Autodesk Fusion 360 part; units mm, degrees
(part 15 of 15)
  spline S61 degree 5 poles (-15.8444, 6.1608) (-15.8425, 6.1587) (-15.8389, 6.1545) (-15.8334, 6.1482) (-15.8261, 6.1398) (-15.8169, 6.1293) (-15.8078, 6.1189) (-15.7986, 6.1086) (-15.7895, 6.0982) (-15.7804, 6.0879) (-15.7712, 6.0777) (-15.7621, 6.0675) (-15.753, 6.0573) (-15.7439, 6.0472) (-15.7347, 6.0371) (-15.7256, 6.027) (-15.7165, 6.017) (-15.7074, 6.007) (-15.6983, 5.9971) (-15.6892, 5.9872) (-15.6801, 5.9774) (-15.671, 5.9676) (-15.6619, 5.9578) (-15.6529, 5.9481) (-15.6438, 5.9384) (-15.6347, 5.9287) (-15.6256, 5.9191) (-15.6166, 5.9096) (-15.6075, 5.9) (-15.5985, 5.8905) (-15.5895, 5.8811) (-15.5804, 5.8717) (-15.5714, 5.8623) (-15.5624, 5.853) (-15.5534, 5.8437) (-15.5444, 5.8345) (-15.5354, 5.8253) (-15.5264, 5.8162) (-15.5174, 5.8071) (-15.5084, 5.798) (-15.4995, 5.789) (-15.4905, 5.78) (-15.4816, 5.771) (-15.4726, 5.7621) (-15.4637, 5.7532) (-15.4548, 5.7444) (-15.4458, 5.7356) (-15.4369, 5.7269) (-15.428, 5.7182) (-15.4192, 5.7096) (-15.4103, 5.7009) (-15.4014, 5.6924) (-15.3926, 5.6838) (-15.3837, 5.6753) (-15.3749, 5.6669) (-15.3661, 5.6585) (-15.3572, 5.6501) (-15.3484, 5.6418) (-15.3397, 5.6335) (-15.3309, 5.6253) (-15.3221, 5.6171) (-15.3134, 5.609) (-15.3046, 5.6008) (-15.2959, 5.5928) (-15.2872, 5.5848) (-15.2785, 5.5768) (-15.2698, 5.5688) (-15.2611, 5.5609) (-15.2524, 5.5531) (-15.2438, 5.5453) (-15.2352, 5.5375) (-15.2265, 5.5298) (-15.2179, 5.5221) (-15.2093, 5.5144) (-15.2008, 5.5068) (-15.1922, 5.4993) (-15.1836, 5.4918) (-15.1751, 5.4843) (-15.1666, 5.4769) (-15.1581, 5.4695) (-15.1496, 5.4621) (-15.1411, 5.4548) (-15.1327, 5.4476) (-15.1242, 5.4403) (-15.1158, 5.4332) (-15.1074, 5.426) (-15.099, 5.419) (-15.0907, 5.4119) (-15.0823, 5.4049) (-15.074, 5.398) (-15.0657, 5.391) (-15.0574, 5.3842) (-15.0491, 5.3773) (-15.0409, 5.3706) (-15.0326, 5.3638) (-15.0244, 5.3571) (-15.0162, 5.3505) (-15.008, 5.3439) (-14.9999, 5.3373) (-14.9918, 5.3308) (-14.9836, 5.3243) (-14.9755, 5.3178) (-14.9675, 5.3114) (-14.9594, 5.3051) (-14.9514, 5.2988) (-14.9434, 5.2925) (-14.9354, 5.2863) (-14.9275, 5.2801) (-14.9195, 5.274) (-14.9116, 5.2679) (-14.9037, 5.2619) (-14.8959, 5.2559) (-14.888, 5.2499) (-14.8802, 5.244) (-14.8724, 5.2381) (-14.8646, 5.2323) (-14.8569, 5.2265) (-14.8492, 5.2208) (-14.8415, 5.2151) (-14.8338, 5.2094) (-14.8262, 5.2038) (-14.8186, 5.1982) (-14.811, 5.1927) (-14.8035, 5.1873) (-14.7959, 5.1818) (-14.7884, 5.1764) (-14.781, 5.1711) (-14.7735, 5.1658) (-14.7661, 5.1605) (-14.7587, 5.1553) (-14.7514, 5.1502) (-14.7441, 5.145) (-14.7368, 5.14) (-14.7295, 5.1349) (-14.7223, 5.1299) (-14.7151, 5.125) (-14.7079, 5.1201) (-14.7008, 5.1152) (-14.6937, 5.1104) (-14.6866, 5.1057) (-14.6796, 5.1009) (-14.6726, 5.0963) (-14.6656, 5.0916) (-14.6587, 5.087) (-14.6518, 5.0825) (-14.6449, 5.078) (-14.6381, 5.0735) (-14.6313, 5.0691) (-14.6245, 5.0648) (-14.6178, 5.0604) (-14.6111, 5.0562) (-14.6045, 5.0519) (-14.5979, 5.0477) (-14.5913, 5.0436) (-14.5848, 5.0395) (-14.5783, 5.0354) (-14.5719, 5.0314) (-14.5655, 5.0275) (-14.5591, 5.0235) (-14.5528, 5.0197) (-14.5465, 5.0158) (-14.5402, 5.0121) (-14.534, 5.0083) (-14.5279, 5.0046) (-14.5218, 5.001) (-14.5157, 4.9974) (-14.5097, 4.9938) (-14.5037, 4.9903) (-14.4978, 4.9868) (-14.4919, 4.9834) (-14.486, 4.98) (-14.4802, 4.9766) (-14.4745, 4.9734) (-14.4688, 4.9701) (-14.4631, 4.9669) (-14.4575, 4.9637) (-14.452, 4.9606) (-14.4465, 4.9576) (-14.441, 4.9545) (-14.4356, 4.9516) (-14.4302, 4.9486) (-14.4249, 4.9457) (-14.4197, 4.9429) (-14.4145, 4.9401) (-14.4094, 4.9373) (-14.4043, 4.9346) (-14.3992, 4.932) (-14.3943, 4.9293) (-14.3894, 4.9268) (-14.3845, 4.9242) (-14.3797, 4.9217) (-14.375, 4.9193) (-14.3703, 4.9169) (-14.3656, 4.9145) (-14.3611, 4.9122) (-14.3566, 4.91) (-14.3521, 4.9078) (-14.3478, 4.9056) (-14.3435, 4.9035) (-14.3392, 4.9014) (-14.335, 4.8993) (-14.3309, 4.8973) (-14.3269, 4.8954) (-14.3229, 4.8935) (-14.319, 4.8916) (-14.3151, 4.8898) (-14.3113, 4.888) (-14.3076, 4.8863) (-14.304, 4.8846) (-14.3004, 4.883) (-14.2969, 4.8814) (-14.2935, 4.8799) (-14.2902, 4.8784) (-14.2869, 4.8769) (-14.2838, 4.8755) (-14.2807, 4.8741) (-14.2776, 4.8728) (-14.2747, 4.8715) (-14.2718, 4.8703) (-14.269, 4.8691) (-14.2663, 4.868) (-14.2637, 4.8669) (-14.2612, 4.8658) (-14.2588, 4.8648) (-14.2564, 4.8638) (-14.2542, 4.8629) (-14.252, 4.862) (-14.2499, 4.8612) (-14.2479, 4.8604) (-14.2461, 4.8596) (-14.2443, 4.8589) (-14.2426, 4.8583) (-14.241, 4.8577) (-14.2395, 4.8571) (-14.2381, 4.8566) (-14.2368, 4.8561) (-14.2356, 4.8556) (-14.2346, 4.8552) (-14.2336, 4.8549) (-14.2328, 4.8546) (-14.232, 4.8543) (-14.2315, 4.8541) (-14.2312, 4.854) (-14.231, 4.8539) (-14.2309, 4.8539) knots -1 -1 -1 -1 -1 -1 -0.99583333 -0.99166667 -0.9875 -0.98333333 -0.97916667 -0.975 -0.97083333 -0.96666667 -0.9625 -0.95833333 -0.95416667 -0.95 -0.94583333 -0.94166667 -0.9375 -0.93333333 -0.92916667 -0.925 -0.92083333 -0.91666667 -0.9125 -0.90833333 -0.90416667 -0.9 -0.89583333 -0.89166667 -0.8875 -0.88333333 -0.87916667 -0.875 -0.87083333 -0.86666667 -0.8625 -0.85833333 -0.85416667 -0.85 -0.84583333 -0.84166667 -0.8375 -0.83333333 -0.82916667 -0.825 -0.82083333 -0.81666667 -0.8125 -0.80833333 -0.80416667 -0.8 -0.79583333 -0.79166667 -0.7875 -0.78333333 -0.77916667 -0.775 -0.77083333 -0.76666667 -0.7625 -0.75833333 -0.75416667 -0.75 -0.74583333 -0.74166667 -0.7375 -0.73333333 -0.72916667 -0.725 -0.72083333 -0.71666667 -0.7125 -0.70833333 -0.70416667 -0.7 -0.69583333 -0.69166667 -0.6875 -0.68333333 -0.67916667 -0.675 -0.67083333 -0.66666667 -0.6625 -0.65833333 -0.65416667 -0.65 -0.64583333 -0.64166667 -0.6375 -0.63333333 -0.62916667 -0.625 -0.62083333 -0.61666667 -0.6125 -0.60833333 -0.60416667 -0.6 -0.59583333 -0.59166667 -0.5875 -0.58333333 -0.57916667 -0.575 -0.57083333 -0.56666667 -0.5625 -0.55833333 -0.55416667 -0.55 -0.54583333 -0.54166667 -0.5375 -0.53333333 -0.52916667 -0.525 -0.52083333 -0.51666667 -0.5125 -0.50833333 -0.50416667 -0.5 -0.49583333 -0.49166667 -0.4875 -0.48333333 -0.47916667 -0.475 -0.47083333 -0.46666667 -0.4625 -0.45833333 -0.45416667 -0.45 -0.44583333 -0.44166667 -0.4375 -0.43333333 -0.42916667 -0.425 -0.42083333 -0.41666667 -0.4125 -0.40833333 -0.40416667 -0.4 -0.39583333 -0.39166667 -0.3875 -0.38333333 -0.37916667 -0.375 -0.37083333 -0.36666667 -0.3625 -0.35833333 -0.35416667 -0.35 -0.34583333 -0.34166667 -0.3375 -0.33333333 -0.32916667 -0.325 -0.32083333 -0.31666667 -0.3125 -0.30833333 -0.30416667 -0.3 -0.29583333 -0.29166667 -0.2875 -0.28333333 -0.27916667 -0.275 -0.27083333 -0.26666667 -0.2625 -0.25833333 -0.25416667 -0.25 -0.24583333 -0.24166667 -0.2375 -0.23333333 -0.22916667 -0.225 -0.22083333 -0.21666667 -0.2125 -0.20833333 -0.20416667 -0.2 -0.19583333 -0.19166667 -0.1875 -0.18333333 -0.17916667 -0.175 -0.17083333 -0.16666667 -0.1625 -0.15833333 -0.15416667 -0.15 -0.14583333 -0.14166667 -0.1375 -0.13333333 -0.12916667 -0.125 -0.12083333 -0.11666667 -0.1125 -0.10833333 -0.10416667 -0.1 -0.09583333 -0.09166667 -0.0875 -0.08333333 -0.07916667 -0.075 -0.07083333 -0.06666667 -0.0625 -0.05833333 -0.05416667 -0.05 -0.04583333 -0.04166667 -0.0375 -0.03333333 -0.02916667 -0.025 -0.02083333 -0.01666667 -0.0125 -0.00833333 -0.00416667 0 0 0 0 0 0
  line L122 (-14.2309, 4.8539) -> (-14.2301, 4.8536)
  line L123 (-14.2301, 4.8536) -> (-13.9603, 4.7616)
  arc A62 (-13.9603, 4.7616) -> (-14.253, 3.7968) centre (0, 0) ccw
  line L124 (-14.253, 3.7968) -> (-14.5284, 3.8702)
  line L125 (-14.5284, 3.8702) -> (-14.5293, 3.8704)
  spline S62 degree 5 poles (-14.5293, 3.8704) (-14.5294, 3.8704) (-14.5296, 3.8705) (-14.5299, 3.8706) (-14.5304, 3.8707) (-14.5312, 3.8709) (-14.532, 3.8711) (-14.533, 3.8713) (-14.5342, 3.8716) (-14.5354, 3.8719) (-14.5367, 3.8722) (-14.5382, 3.8725) (-14.5397, 3.8729) (-14.5414, 3.8733) (-14.5432, 3.8736) (-14.545, 3.874) (-14.547, 3.8745) (-14.5491, 3.8749) (-14.5513, 3.8754) (-14.5536, 3.8758) (-14.556, 3.8763) (-14.5585, 3.8768) (-14.5611, 3.8773) (-14.5637, 3.8779) (-14.5665, 3.8784) (-14.5694, 3.8789) (-14.5724, 3.8795) (-14.5754, 3.8801) (-14.5786, 3.8806) (-14.5818, 3.8812) (-14.5852, 3.8818) (-14.5886, 3.8824) (-14.5921, 3.883) (-14.5957, 3.8836) (-14.5994, 3.8842) (-14.6032, 3.8848) (-14.6071, 3.8854) (-14.6111, 3.8861) (-14.6151, 3.8867) (-14.6192, 3.8873) (-14.6234, 3.8879) (-14.6277, 3.8886) (-14.6321, 3.8892) (-14.6365, 3.8898) (-14.6411, 3.8905) (-14.6457, 3.8911) (-14.6504, 3.8917) (-14.6551, 3.8923) (-14.66, 3.893) (-14.6649, 3.8936) (-14.6699, 3.8942) (-14.675, 3.8948) (-14.6801, 3.8954) (-14.6854, 3.8961) (-14.6907, 3.8967) (-14.696, 3.8973) (-14.7015, 3.8979) (-14.707, 3.8984) (-14.7126, 3.899) (-14.7182, 3.8996) (-14.724, 3.9002) (-14.7298, 3.9007) (-14.7357, 3.9013) (-14.7416, 3.9018) (-14.7476, 3.9024) (-14.7537, 3.9029) (-14.7598, 3.9034) (-14.7661, 3.904) (-14.7723, 3.9045) (-14.7787, 3.905) (-14.7851, 3.9054) (-14.7916, 3.9059) (-14.7981, 3.9064) (-14.8047, 3.9068) (-14.8114, 3.9073) (-14.8182, 3.9077) (-14.825, 3.9081) (-14.8318, 3.9086) (-14.8388, 3.909) (-14.8457, 3.9093) (-14.8528, 3.9097) (-14.8599, 3.9101) (-14.8671, 3.9104) (-14.8743, 3.9108) (-14.8816, 3.9111) (-14.889, 3.9114) (-14.8964, 3.9117) (-14.9038, 3.912) (-14.9114, 3.9122) (-14.919, 3.9125) (-14.9266, 3.9127) (-14.9343, 3.9129) (-14.9421, 3.9131) (-14.9499, 3.9133) (-14.9578, 3.9135) (-14.9657, 3.9136) (-14.9737, 3.9138) (-14.9817, 3.9139) (-14.9898, 3.914) (-14.998, 3.9141) (-15.0062, 3.9141) (-15.0145, 3.9142) (-15.0228, 3.9142) (-15.0311, 3.9143) (-15.0396, 3.9143) (-15.048, 3.9142) (-15.0565, 3.9142) (-15.0651, 3.9141) (-15.0738, 3.9141) (-15.0824, 3.914) (-15.0912, 3.9139) (-15.0999, 3.9137) (-15.1088, 3.9136) (-15.1177, 3.9134) (-15.1266, 3.9132) (-15.1356, 3.913) (-15.1446, 3.9128) (-15.1537, 3.9125) (-15.1628, 3.9123) (-15.172, 3.912) (-15.1812, 3.9116) (-15.1905, 3.9113) (-15.1998, 3.911) (-15.2092, 3.9106) (-15.2186, 3.9102) (-15.2281, 3.9098) (-15.2376, 3.9093) (-15.2471, 3.9089) (-15.2568, 3.9084) (-15.2664, 3.9079) (-15.2761, 3.9073) (-15.2858, 3.9068) (-15.2956, 3.9062) (-15.3054, 3.9056) (-15.3153, 3.905) (-15.3252, 3.9043) (-15.3352, 3.9037) (-15.3452, 3.903) (-15.3553, 3.9023) (-15.3653, 3.9015) (-15.3755, 3.9008) (-15.3857, 3.9) (-15.3959, 3.8992) (-15.4061, 3.8983) (-15.4164, 3.8975) (-15.4268, 3.8966) (-15.4372, 3.8957) (-15.4476, 3.8948) (-15.4581, 3.8938) (-15.4686, 3.8928) (-15.4791, 3.8918) (-15.4897, 3.8908) (-15.5004, 3.8897) (-15.511, 3.8887) (-15.5218, 3.8876) (-15.5325, 3.8864) (-15.5433, 3.8853) (-15.5541, 3.8841) (-15.565, 3.8829) (-15.5759, 3.8816) (-15.5869, 3.8804) (-15.5978, 3.8791) (-15.6089, 3.8778) (-15.6199, 3.8764) (-15.631, 3.8751) (-15.6422, 3.8737) (-15.6533, 3.8723) (-15.6645, 3.8708) (-15.6758, 3.8693) (-15.6871, 3.8678) (-15.6984, 3.8663) (-15.7097, 3.8648) (-15.7211, 3.8632) (-15.7326, 3.8616) (-15.744, 3.8599) (-15.7555, 3.8583) (-15.7671, 3.8566) (-15.7786, 3.8549) (-15.7902, 3.8531) (-15.8019, 3.8513) (-15.8135, 3.8495) (-15.8252, 3.8477) (-15.837, 3.8459) (-15.8488, 3.844) (-15.8606, 3.8421) (-15.8724, 3.8401) (-15.8843, 3.8381) (-15.8962, 3.8361) (-15.9081, 3.8341) (-15.9201, 3.8321) (-15.9321, 3.83) (-15.9441, 3.8279) (-15.9562, 3.8257) (-15.9683, 3.8235) (-15.9805, 3.8213) (-15.9926, 3.8191) (-16.0048, 3.8168) (-16.017, 3.8146) (-16.0293, 3.8122) (-16.0416, 3.8099) (-16.0539, 3.8075) (-16.0663, 3.8051) (-16.0786, 3.8027) (-16.0911, 3.8002) (-16.1035, 3.7977) (-16.116, 3.7952) (-16.1285, 3.7926) (-16.141, 3.79) (-16.1536, 3.7874) (-16.1661, 3.7848) (-16.1788, 3.7821) (-16.1914, 3.7794) (-16.2041, 3.7766) (-16.2168, 3.7739) (-16.2295, 3.7711) (-16.2423, 3.7683) (-16.2551, 3.7654) (-16.2679, 3.7625) (-16.2807, 3.7596) (-16.2936, 3.7566) (-16.3065, 3.7536) (-16.3194, 3.7506) (-16.3324, 3.7476) (-16.3454, 3.7445) (-16.3584, 3.7414) (-16.3714, 3.7383) (-16.3845, 3.7351) (-16.3976, 3.7319) (-16.4107, 3.7287) (-16.4238, 3.7254) (-16.437, 3.7221) (-16.4502, 3.7188) (-16.4634, 3.7154) (-16.4766, 3.712) (-16.4899, 3.7086) (-16.5032, 3.7052) (-16.5165, 3.7017) (-16.5298, 3.6982) (-16.5432, 3.6946) (-16.5566, 3.691) (-16.57, 3.6874) (-16.5807, 3.6845) (-16.5888, 3.6823) (-16.5942, 3.6808) (-16.5969, 3.6801) knots 0 0 0 0 0 0 0.00416667 0.00833333 0.0125 0.01666667 0.02083333 0.025 0.02916667 0.03333333 0.0375 0.04166667 0.04583333 0.05 0.05416667 0.05833333 0.0625 0.06666667 0.07083333 0.075 0.07916667 0.08333333 0.0875 0.09166667 0.09583333 0.1 0.10416667 0.10833333 0.1125 0.11666667 0.12083333 0.125 0.12916667 0.13333333 0.1375 0.14166667 0.14583333 0.15 0.15416667 0.15833333 0.1625 0.16666667 0.17083333 0.175 0.17916667 0.18333333 0.1875 0.19166667 0.19583333 0.2 0.20416667 0.20833333 0.2125 0.21666667 0.22083333 0.225 0.22916667 0.23333333 0.2375 0.24166667 0.24583333 0.25 0.25416667 0.25833333 0.2625 0.26666667 0.27083333 0.275 0.27916667 0.28333333 0.2875 0.29166667 0.29583333 0.3 0.30416667 0.30833333 0.3125 0.31666667 0.32083333 0.325 0.32916667 0.33333333 0.3375 0.34166667 0.34583333 0.35 0.35416667 0.35833333 0.3625 0.36666667 0.37083333 0.375 0.37916667 0.38333333 0.3875 0.39166667 0.39583333 0.4 0.40416667 0.40833333 0.4125 0.41666667 0.42083333 0.425 0.42916667 0.43333333 0.4375 0.44166667 0.44583333 0.45 0.45416667 0.45833333 0.4625 0.46666667 0.47083333 0.475 0.47916667 0.48333333 0.4875 0.49166667 0.49583333 0.5 0.50416667 0.50833333 0.5125 0.51666667 0.52083333 0.525 0.52916667 0.53333333 0.5375 0.54166667 0.54583333 0.55 0.55416667 0.55833333 0.5625 0.56666667 0.57083333 0.575 0.57916667 0.58333333 0.5875 0.59166667 0.59583333 0.6 0.60416667 0.60833333 0.6125 0.61666667 0.62083333 0.625 0.62916667 0.63333333 0.6375 0.64166667 0.64583333 0.65 0.65416667 0.65833333 0.6625 0.66666667 0.67083333 0.675 0.67916667 0.68333333 0.6875 0.69166667 0.69583333 0.7 0.70416667 0.70833333 0.7125 0.71666667 0.72083333 0.725 0.72916667 0.73333333 0.7375 0.74166667 0.74583333 0.75 0.75416667 0.75833333 0.7625 0.76666667 0.77083333 0.775 0.77916667 0.78333333 0.7875 0.79166667 0.79583333 0.8 0.80416667 0.80833333 0.8125 0.81666667 0.82083333 0.825 0.82916667 0.83333333 0.8375 0.84166667 0.84583333 0.85 0.85416667 0.85833333 0.8625 0.86666667 0.87083333 0.875 0.87916667 0.88333333 0.8875 0.89166667 0.89583333 0.9 0.90416667 0.90833333 0.9125 0.91666667 0.92083333 0.925 0.92916667 0.93333333 0.9375 0.94166667 0.94583333 0.95 0.95416667 0.95833333 0.9625 0.96666667 0.97083333 0.975 0.97916667 0.98333333 0.9875 0.99166667 0.99583333 1 1 1 1 1 1
  arc A63 (-16.5969, 3.6801) -> (-16.7418, 2.9514) centre (0, 0) ccw
  spline S63 degree 5 poles (-16.7418, 2.9514) (-16.7396, 2.9497) (-16.7352, 2.9462) (-16.7286, 2.9411) (-16.7198, 2.9343) (-16.7088, 2.9258) (-16.6978, 2.9174) (-16.6868, 2.909) (-16.6758, 2.9007) (-16.6648, 2.8924) (-16.6539, 2.8841) (-16.6429, 2.8758) (-16.632, 2.8676) (-16.6211, 2.8595) (-16.6102, 2.8514) (-16.5993, 2.8433) (-16.5884, 2.8352) (-16.5775, 2.8272) (-16.5666, 2.8193) (-16.5558, 2.8114) (-16.5449, 2.8035) (-16.5341, 2.7956) (-16.5233, 2.7878) (-16.5125, 2.78) (-16.5017, 2.7723) (-16.4909, 2.7646) (-16.4802, 2.757) (-16.4694, 2.7494) (-16.4587, 2.7418) (-16.448, 2.7342) (-16.4373, 2.7267) (-16.4266, 2.7193) (-16.4159, 2.7119) (-16.4052, 2.7045) (-16.3946, 2.6971) (-16.3839, 2.6898) (-16.3733, 2.6826) (-16.3627, 2.6754) (-16.3521, 2.6682) (-16.3416, 2.661) (-16.331, 2.6539) (-16.3205, 2.6469) (-16.3099, 2.6398) (-16.2994, 2.6328) (-16.289, 2.6259) (-16.2785, 2.619) (-16.268, 2.6121) (-16.2576, 2.6053) (-16.2472, 2.5985) (-16.2368, 2.5917) (-16.2264, 2.585) (-16.216, 2.5783) (-16.2057, 2.5717) (-16.1953, 2.5651) (-16.185, 2.5585) (-16.1747, 2.552) (-16.1645, 2.5455) (-16.1542, 2.5391) (-16.144, 2.5327) (-16.1337, 2.5263) (-16.1235, 2.52) (-16.1134, 2.5137) (-16.1032, 2.5074) (-16.0931, 2.5012) (-16.083, 2.4951) (-16.0729, 2.4889) (-16.0628, 2.4828) (-16.0527, 2.4768) (-16.0427, 2.4708) (-16.0327, 2.4648) (-16.0227, 2.4589) (-16.0128, 2.453) (-16.0028, 2.4471) (-15.9929, 2.4413) (-15.983, 2.4355) (-15.9731, 2.4298) (-15.9633, 2.4241) (-15.9535, 2.4184) (-15.9436, 2.4128) (-15.9339, 2.4072) (-15.9241, 2.4016) (-15.9144, 2.3961) (-15.9047, 2.3907) (-15.895, 2.3852) (-15.8853, 2.3798) (-15.8757, 2.3745) (-15.8661, 2.3692) (-15.8565, 2.3639) (-15.847, 2.3586) (-15.8374, 2.3534) (-15.8279, 2.3483) (-15.8185, 2.3432) (-15.809, 2.3381) (-15.7996, 2.333) (-15.7902, 2.328) (-15.7808, 2.3231) (-15.7715, 2.3181) (-15.7622, 2.3132) (-15.7529, 2.3084) (-15.7437, 2.3036) (-15.7344, 2.2988) (-15.7253, 2.2941) (-15.7161, 2.2894) (-15.707, 2.2847) (-15.6979, 2.2801) (-15.6888, 2.2755) (-15.6797, 2.271) (-15.6707, 2.2665) (-15.6617, 2.262) (-15.6528, 2.2576) (-15.6439, 2.2532) (-15.635, 2.2488) (-15.6261, 2.2445) (-15.6173, 2.2402) (-15.6085, 2.236) (-15.5998, 2.2318) (-15.5911, 2.2276) (-15.5824, 2.2235) (-15.5737, 2.2194) (-15.5651, 2.2154) (-15.5565, 2.2114) (-15.548, 2.2074) (-15.5395, 2.2035) (-15.531, 2.1996) (-15.5226, 2.1957) (-15.5141, 2.1919) (-15.5058, 2.1881) (-15.4974, 2.1844) (-15.4892, 2.1807) (-15.4809, 2.177) (-15.4727, 2.1734) (-15.4645, 2.1698) (-15.4564, 2.1662) (-15.4483, 2.1627) (-15.4402, 2.1592) (-15.4322, 2.1558) (-15.4242, 2.1523) (-15.4162, 2.149) (-15.4083, 2.1456) (-15.4005, 2.1423) (-15.3927, 2.1391) (-15.3849, 2.1359) (-15.3771, 2.1327) (-15.3694, 2.1295) (-15.3618, 2.1264) (-15.3542, 2.1233) (-15.3466, 2.1203) (-15.3391, 2.1173) (-15.3316, 2.1143) (-15.3242, 2.1114) (-15.3168, 2.1085) (-15.3095, 2.1057) (-15.3022, 2.1028) (-15.2949, 2.1001) (-15.2877, 2.0973) (-15.2806, 2.0946) (-15.2735, 2.0919) (-15.2664, 2.0893) (-15.2594, 2.0867) (-15.2524, 2.0841) (-15.2455, 2.0816) (-15.2387, 2.0791) (-15.2318, 2.0766) (-15.2251, 2.0742) (-15.2184, 2.0718) (-15.2117, 2.0695) (-15.2051, 2.0671) (-15.1986, 2.0649) (-15.1921, 2.0626) (-15.1856, 2.0604) (-15.1792, 2.0582) (-15.1729, 2.0561) (-15.1666, 2.054) (-15.1604, 2.0519) (-15.1542, 2.0499) (-15.1481, 2.0478) (-15.142, 2.0459) (-15.136, 2.0439) (-15.1301, 2.042) (-15.1242, 2.0402) (-15.1184, 2.0383) (-15.1126, 2.0365) (-15.1069, 2.0348) (-15.1013, 2.033) (-15.0957, 2.0313) (-15.0902, 2.0297) (-15.0847, 2.028) (-15.0794, 2.0264) (-15.074, 2.0249) (-15.0688, 2.0233) (-15.0636, 2.0218) (-15.0584, 2.0204) (-15.0534, 2.0189) (-15.0484, 2.0175) (-15.0435, 2.0161) (-15.0386, 2.0148) (-15.0338, 2.0135) (-15.0291, 2.0122) (-15.0245, 2.011) (-15.0199, 2.0098) (-15.0154, 2.0086) (-15.011, 2.0074) (-15.0066, 2.0063) (-15.0023, 2.0052) (-14.9981, 2.0042) (-14.994, 2.0031) (-14.99, 2.0021) (-14.986, 2.0012) (-14.9821, 2.0002) (-14.9783, 1.9993) (-14.9746, 1.9984) (-14.9709, 1.9976) (-14.9673, 1.9968) (-14.9639, 1.996) (-14.9605, 1.9952) (-14.9571, 1.9945) (-14.9539, 1.9937) (-14.9508, 1.9931) (-14.9477, 1.9924) (-14.9448, 1.9918) (-14.9419, 1.9912) (-14.9391, 1.9906) (-14.9365, 1.9901) (-14.9339, 1.9896) (-14.9314, 1.9891) (-14.929, 1.9886) (-14.9267, 1.9882) (-14.9245, 1.9877) (-14.9224, 1.9874) (-14.9204, 1.987) (-14.9185, 1.9866) (-14.9167, 1.9863) (-14.915, 1.986) (-14.9135, 1.9858) (-14.912, 1.9855) (-14.9106, 1.9853) (-14.9094, 1.9851) (-14.9083, 1.9849) (-14.9073, 1.9848) (-14.9064, 1.9846) (-14.9056, 1.9845) (-14.9051, 1.9844) (-14.9047, 1.9844) (-14.9045, 1.9843) (-14.9044, 1.9843) knots -1 -1 -1 -1 -1 -1 -0.99583333 -0.99166667 -0.9875 -0.98333333 -0.97916667 -0.975 -0.97083333 -0.96666667 -0.9625 -0.95833333 -0.95416667 -0.95 -0.94583333 -0.94166667 -0.9375 -0.93333333 -0.92916667 -0.925 -0.92083333 -0.91666667 -0.9125 -0.90833333 -0.90416667 -0.9 -0.89583333 -0.89166667 -0.8875 -0.88333333 -0.87916667 -0.875 -0.87083333 -0.86666667 -0.8625 -0.85833333 -0.85416667 -0.85 -0.84583333 -0.84166667 -0.8375 -0.83333333 -0.82916667 -0.825 -0.82083333 -0.81666667 -0.8125 -0.80833333 -0.80416667 -0.8 -0.79583333 -0.79166667 -0.7875 -0.78333333 -0.77916667 -0.775 -0.77083333 -0.76666667 -0.7625 -0.75833333 -0.75416667 -0.75 -0.74583333 -0.74166667 -0.7375 -0.73333333 -0.72916667 -0.725 -0.72083333 -0.71666667 -0.7125 -0.70833333 -0.70416667 -0.7 -0.69583333 -0.69166667 -0.6875 -0.68333333 -0.67916667 -0.675 -0.67083333 -0.66666667 -0.6625 -0.65833333 -0.65416667 -0.65 -0.64583333 -0.64166667 -0.6375 -0.63333333 -0.62916667 -0.625 -0.62083333 -0.61666667 -0.6125 -0.60833333 -0.60416667 -0.6 -0.59583333 -0.59166667 -0.5875 -0.58333333 -0.57916667 -0.575 -0.57083333 -0.56666667 -0.5625 -0.55833333 -0.55416667 -0.55 -0.54583333 -0.54166667 -0.5375 -0.53333333 -0.52916667 -0.525 -0.52083333 -0.51666667 -0.5125 -0.50833333 -0.50416667 -0.5 -0.49583333 -0.49166667 -0.4875 -0.48333333 -0.47916667 -0.475 -0.47083333 -0.46666667 -0.4625 -0.45833333 -0.45416667 -0.45 -0.44583333 -0.44166667 -0.4375 -0.43333333 -0.42916667 -0.425 -0.42083333 -0.41666667 -0.4125 -0.40833333 -0.40416667 -0.4 -0.39583333 -0.39166667 -0.3875 -0.38333333 -0.37916667 -0.375 -0.37083333 -0.36666667 -0.3625 -0.35833333 -0.35416667 -0.35 -0.34583333 -0.34166667 -0.3375 -0.33333333 -0.32916667 -0.325 -0.32083333 -0.31666667 -0.3125 -0.30833333 -0.30416667 -0.3 -0.29583333 -0.29166667 -0.2875 -0.28333333 -0.27916667 -0.275 -0.27083333 -0.26666667 -0.2625 -0.25833333 -0.25416667 -0.25 -0.24583333 -0.24166667 -0.2375 -0.23333333 -0.22916667 -0.225 -0.22083333 -0.21666667 -0.2125 -0.20833333 -0.20416667 -0.2 -0.19583333 -0.19166667 -0.1875 -0.18333333 -0.17916667 -0.175 -0.17083333 -0.16666667 -0.1625 -0.15833333 -0.15416667 -0.15 -0.14583333 -0.14166667 -0.1375 -0.13333333 -0.12916667 -0.125 -0.12083333 -0.11666667 -0.1125 -0.10833333 -0.10416667 -0.1 -0.09583333 -0.09166667 -0.0875 -0.08333333 -0.07916667 -0.075 -0.07083333 -0.06666667 -0.0625 -0.05833333 -0.05416667 -0.05 -0.04583333 -0.04166667 -0.0375 -0.03333333 -0.02916667 -0.025 -0.02083333 -0.01666667 -0.0125 -0.00833333 -0.00416667 0 0 0 0 0 0
  line L126 (-14.9044, 1.9843) -> (-14.9036, 1.9842)
  line L127 (-14.9036, 1.9842) -> (-14.621, 1.9466)
  circle A64 centre (0, 0) radius 10
  circle A65 centre (0, 0) radius 3
  dimension "d7" = 20
  dimension "d8" = 6
  constraint concentric A0 A64
  constraint concentric A64 A65
  measures "d7" diameter of A64
  measures "d8" diameter of A65
extrude "Extrude3" add sketch "Sketch1 (2)" along normal blind 8.1 contours A64 bodies 1 in component "Component"
extrude "Extrude4" cut sketch "Sketch1 (2)" against normal blind 10 contours A65 bodies 1 in component "Component"
component "Component" placed x (1, 0, 0) y (0, 1, 0) z (0, 0, 1) at (0, 0, 0)
